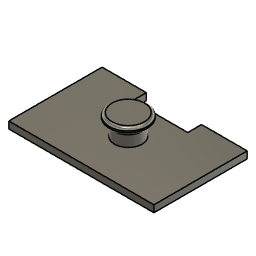
Rpi lid v6 (Autodesk Fusion 360 design; units mm, degrees)
Autodesk Fusion 360 part; units mm, degrees
sketch "Sketch1" plane through (0, 0, 0) normal (0, 1, 0) x (1, 0, 0)
  line L0 (0, 0) -> (105.3, 0)
  line L1 (105.3, 0) -> (105.3, -67.7)
  line L2 (105.3, -67.7) -> (0, -67.7)
  line L3 (0, -67.7) -> (0, 0)
  dimension "d1" = 105.3
  dimension "d2" = 67.7
  constraint horizontal L0
  constraint vertical L1
  constraint horizontal L2
  constraint vertical L3
  constraint coincident L0.start L3.end
  measures "d1" distance of L0.start L0.end
  measures "d2" distance of L0.start L2.end
extrude "Extrude1" add sketch "Sketch1" along normal blind 5 makes body 1
sketch "Sketch2" plane through (0, 5, 0) normal (0, 1, 0) x (-1, 0, 0)
  line L0 (0, 67.7) -> (-105.3, 67.7)
  line L1 (-105.3, 67.7) -> (-105.3, 0)
  line L2 (-105.3, 0) -> (0, 0)
  line L3 (0, 0) -> (0, 67.7)
  line L4 (-52.65, 0) -> (-52.65, 67.7)
  line L5 (-26.1, 0) -> (-26.1, 68.1)
  line L6 (-74.6077, 28.85) -> (-84.6077, 28.85)
  line L7 (-84.6077, 28.85) -> (-84.6077, 38.85)
  line L8 (-84.6077, 38.85) -> (-74.6077, 38.85)
  line L9 (-74.6077, 38.85) -> (-74.6077, 28.85)
  line L10 (-20.6923, 28.85) -> (-20.6923, 38.85)
  line L11 (-20.6923, 38.85) -> (-30.6923, 38.85)
  line L12 (-30.6923, 28.85) -> (-20.6923, 28.85)
  line L13 (-30.6923, 38.85) -> (-30.6923, 28.85)
  dimension "d8" = 10
  dimension "d9" = 10
  constraint midpoint L2 L4.start
  constraint midpoint L0 L4.end
  constraint horizontal L6
  constraint vertical L7
  constraint horizontal L8
  constraint vertical L9
  constraint symmetric L4 L6.start L12.start
  constraint symmetric L4 L6.end L10.start
  constraint symmetric L4 L7.end L10.end
  constraint symmetric L4 L8.end L11.end
  measures "d8" distance of L6.start L6.end
  measures "d9" distance of L6.start L8.end
revolve "Revolve1" add sketch "Sketch2" angle 180 about axis through (52.65, 5, 0) along (0, 0, 1) contours L6 L7 L8 L9 bodies 1
copy_body "CopyPasteBodies1" bodies 1 makes body 2
delete_face "DeleteFace1" 1 faces at (39.7723, 30.4802, 28.85) on bodies 1
delete_face "DeleteFace2" 1 faces at (20.732, 6.593, 32.1833) on bodies 2
sketch "Sketch3" plane through (0, 5, 0) normal (0, 1, 0) x (-1, 0, 0)
  line L0 (-105.3, 0) -> (0, 0)
  line L1 (0, 0) -> (0, 67.7)
  line L2 (0, 67.7) -> (-105.3, 67.7)
  line L3 (-105.3, 67.7) -> (-105.3, 0)
  circle A0 centre (-52.95, 33.95) radius 10
  dimension "d11" = 20
  measures "d11" diameter of A0
extrude "Extrude2" add sketch "Sketch3" along normal blind 10 contours A0 bodies 1 2
sketch "Sketch4" plane through (0, 15, 0) normal (0, 1, 0) x (-1, 0, 0)
  circle A0 centre (-52.95, 33.95) radius 10
  circle A1 centre (-52.95, 33.95) radius 13.7989
  constraint concentric A0 A1
extrude "Extrude3" add sketch "Sketch4" along normal blind 5 contours A0 | A1 bodies 1
fillet "Fillet1" radius 2 tangency weight 1.37089 1 edges at (62.2733, 15, 30.3338) on bodies 1
fillet "Fillet2" radius 2 2 edges at (65.8151, 20, 28.9601) (65.8151, 15, 28.9601) on bodies 1
sketch "Sketch5" plane through (0, 5, 0) normal (0, 1, 0) x (-1, 0, 0)
  circle A0 centre (-52.95, 33.95) radius 10
  line L0 (-105.3, 0) -> (0, 0)
  line L1 (0, 0) -> (0, 67.7)
  line L2 (0, 67.7) -> (-105.3, 67.7)
  line L3 (-105.3, 67.7) -> (-105.3, 0)
  line L4 (-32.1296, 0) -> (-72.1296, 0)
  line L5 (-72.1296, 0) -> (-72.1296, 10)
  line L6 (-72.1296, 10) -> (-32.1296, 10)
  line L7 (-32.1296, 10) -> (-32.1296, 0)
  constraint horizontal L4
  constraint vertical L5
  constraint horizontal L6
  constraint vertical L7
  constraint coincident L0 L4.start
extrude "Extrude4" cut sketch "Sketch5" against normal blind 10 contours L0 L4 L5 L6 L7 bodies 1
